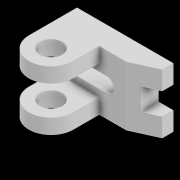
# Autodesk Inventor part: 零件2
Saved by Autodesk Inventor 2020 (Build 240168000, 168)
## iProperties
Created: 2020-11-12
Part Number: 零件2
Material: 常规
Document SubType Name: Modeling
Designer: NH55
Density: 1 g/cm^3
Appearance: 默认
Author: NH55
Autodesk Inventor part; units mm, degrees
ref_plane "YZ Plane" through (0, 0, 0) normal (1, 0, 0) x (0, 1, 0)
ref_plane "XZ Plane" through (0, 0, 0) normal (0, 1, 0) x (-1, 0, 0)
ref_plane "XY Plane" through (0, 0, 0) normal (0, 0, 1) x (1, 0, 0)
sketch "草图2" plane through (0, 0, 0) normal (0, 1, 0) x (-1, 0, 0)
  line L0 (29.7873, 9.5105) -> (-28.2127, 9.5105)
  line L1 (-28.2127, 9.5105) -> (-48.2127, 0.5105)
  line L2 (-48.2127, 0.5105) -> (-48.2127, -8.4895)
  line L3 (-48.2127, -8.4895) -> (29.7873, -8.4895)
  line L4 (29.7873, -8.4895) -> (29.7873, 9.5105)
  dimension "d3" = 9
  dimension "d4" = 78
  dimension "d5" = 18
  dimension "d6" = 58
  constraints: 10 end point, 3 perpendicular, 1 horizontal
  measures "d3" distance of L1.end L2.end
  measures "d4" distance of L2.end L3.end
  measures "d5" distance of L3.end L0.start
  measures "d6" distance of L0.start L0.end
extrude "拉伸1" add sketch "草图2" along normal mid plane 48
sketch "草图3" plane through (48.2127, 24, -8.4895) normal (0, 0, -1) x (-1, 0, 0)
  line L0 (78, -48) -> (78, 0) projected
  line L1 (0, 0) -> (78, 0) projected
  line L2 (0, -48) -> (0, 0) projected
  line L3 (78, -48) -> (0, -48) projected
  line L4 (0, -48) -> (0, 0) projected
  line L5 (0, -33) -> (12, -33)
  line L6 (12, -33) -> (12, -15)
  line L7 (12, -15) -> (0, -15)
  line L8 (0, -15) -> (0, -33)
  point P0 (48.2127, -24)
  point P1 (0, -24)
  point P2 (0, -24)
  point P3 (0, -24)
  dimension "d9" = 18
  dimension "d10" = 12
  constraints: 8 end point, 3 midpoint, 2 coincident, 2 perpendicular, 2 point on line, 1 collinear, 1 horizontal
  measures "d9" distance of L5.end L6.end
  measures "d10" distance of L6.end L7.end
extrude "拉伸2" cut sketch "草图3" against normal up to surface contours L2 L7 L6 L5 surface through (28.2127, 0, 9.5105) normal (0.4103647, 0, 0.9119215)
sketch "草图4" plane through (0, 24, 0) normal (0, 1, 0) x (1, 0, 0)
  line L0 (28.2127, -9.5105) -> (48.2127, -0.5105) projected
  line L1 (48.2127, -0.5105) -> (48.2127, 8.4895) projected
  line L2 (48.2127, 8.4895) -> (-29.7873, 8.4895) projected
  line L3 (-29.7873, 8.4895) -> (-29.7873, -9.5105) projected
  line L4 (-29.7873, -9.5105) -> (28.2127, -9.5105) projected
  line L5 (28.2127, -9.5105) -> (-29.7873, -9.5105) projected
  line L6 (-29.7873, -9.5105) -> (-29.7873, -30.5105)
  arc A0 (-29.7873, -30.5105) -> (6.2127, -30.5105) centre (-11.7873, -30.5105) ccw
  line L7 (6.2127, -30.5105) -> (6.2127, -9.5105)
  circle A1 centre (-11.7873, -30.5105) radius 9
  point P0 (0, 0)
  dimension "d13" = 39
  dimension "d14" = 18
  dimension "d15" = 18
  constraints: 4 end point, 2 centre point, 2 point on circle, 2 tangent, 1 coincident, 1 perpendicular, 1 point on line, 1 vertical
  measures "d13" distance from line of L2 A0.centre
  measures "d14" radius of A0
  measures "d15" diameter of A1
extrude "拉伸3" add sketch "草图4" against normal blind 12 contours L7 A0 L6 L4
mirror "镜像1" about plane through (0, 0, 0) normal (0, 1, 0) of "拉伸3"
sketch "草图5" plane through (28.2127, -24, 9.5105) normal (0, 0, 1) x (1, 0, 0)
  line L0 (-58, 12) -> (-22, 12) projected
  line L1 (-22, 12) -> (-22, 0) projected
  line L2 (0, 0) -> (-22, 0) projected
  line L3 (0, 48) -> (0, 0) projected
  line L4 (-22, 48) -> (0, 48) projected
  line L5 (-22, 48) -> (-22, 36) projected
  line L6 (-22, 36) -> (-58, 36) projected
  line L7 (-58, 12) -> (-58, 36) projected
  line L8 (-16, 18) -> (-43, 18)
  arc A0 (-43, 30) -> (-43, 18) centre (-43, 24) ccw
  line L9 (-43, 30) -> (-16, 30)
  arc A1 (-16, 18) -> (-16, 30) centre (-16, 24) ccw
  point P0 (-28.2127, 24)
  point P1 (-58, 24)
  dimension "d18" = 6
  dimension "d19" = 27
  dimension "d20" = 15
  constraints: 4 end point, 4 point on circle, 4 tangent, 2 centre point, 1 horizontal, 1 horizontal alignment, 1 midpoint, 1 parallel
  measures "d18" radius of A0
  measures "d19" distance of L8.start L8.end
  measures "d20" distance from line of L7 A0.centre
extrude "拉伸4" cut sketch "草图5" against normal up to surface (18 mm away) contours L8 A0 L9 A1
